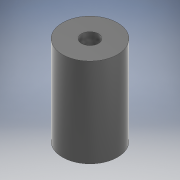
# Autodesk Inventor part: coupling_encoder
Saved by Autodesk Inventor 2022 (Build 260153070, 153G)
## iProperties
Created: 2020-10-29
Part Number: coupling_encoder
Material: ABS プラスチック
Document SubType Name: Modeling
Designer: Haruka
Density: 1.06 g/cm^3
Appearance: 滑らか - 黒
Author: Haruka
Autodesk Inventor part; units mm, degrees
ref_plane "YZ Plane" through (0, 0, 0) normal (1, 0, 0) x (0, 1, 0)
ref_plane "XZ Plane" through (0, 0, 0) normal (0, 1, 0) x (-1, 0, 0)
ref_plane "XY Plane" through (0, 0, 0) normal (0, 0, 1) x (1, 0, 0)
sketch "スケッチ1" plane through (0, 0, 0) normal (0, 1, 0) x (-1, 0, 0)
  circle A0 centre (0, 0) radius 6.5
  circle A1 centre (0, 0) radius 2
  dimension "d0" = 13
  dimension "d1" = 4
  constraints: 2 centre point, 2 coincident
  measures "d0" diameter of A0
  measures "d1" diameter of A1
extrude "押し出し1" add sketch "スケッチ1" along normal blind 21
